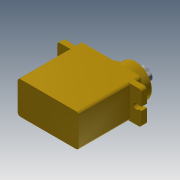
# Autodesk Inventor part: micro_servo
Saved by Autodesk Inventor 2015 (Build 190159000, 159)
## iProperties
Created: 2013-01-22
Part Number: micro_servo
Material: Generic
Document SubType Name: Modeling
Designer: idle-rug
Density: 1 g/cm^3
Appearance: Default
Author: idle-rug
Autodesk Inventor part; units mm, degrees
ref_plane "YZ Plane" through (0, 0, 0) normal (1, 0, 0) x (0, 1, 0)
ref_plane "XZ Plane" through (0, 0, 0) normal (0, 1, 0) x (-1, 0, 0)
ref_plane "XY Plane" through (0, 0, 0) normal (0, 0, 1) x (1, 0, 0)
sketch "Sketch1" plane through (0, 0, 0) normal (0, 1, 0) x (-1, 0, 0)
  line L0 (-11.6, -6.2) -> (11.6, -6.2)
  line L1 (11.6, -6.2) -> (11.6, 6.2)
  line L2 (11.6, 6.2) -> (-11.6, 6.2)
  line L3 (-11.6, 6.2) -> (-11.6, -6.2)
  line L4 (-11.6, -6.2) -> (11.6, 6.2) construction
  line L5 (11.6, -6.2) -> (-11.6, 6.2) construction
  point P0 (0, 0)
  constraints: 12 end point, 2 midpoint, 2 parallel, 1 horizontal, 1 perpendicular
extrude "Extrusion1" add sketch "Sketch1" along normal blind 31.7
sketch "Sketch2" plane through (11.6, 0, 6.2) normal (1, 0, 0) x (0, 0, -1)
  line L0 (12.4, 19.4) -> (0, 19.4)
  line L1 (0, 19.4) -> (0, 21.5)
  line L2 (0, 21.5) -> (12.4, 21.5)
  line L3 (12.4, 21.5) -> (12.4, 19.4)
  constraints: 8 end point
extrude "Extrusion2" add sketch "Sketch2" along normal blind 4.4
sketch "Sketch8" plane through (-11.6, 0, -6.2) normal (-1, 0, 0) x (0, 0, 1)
  line L0 (12.4, 19.4) -> (0, 19.4)
  line L1 (0, 19.4) -> (0, 21.5)
  line L2 (0, 21.5) -> (12.4, 21.5)
  line L3 (12.4, 21.5) -> (12.4, 19.4)
  point P0 (12.4, 0)
  point P1 (6.2, 0)
  constraints: 8 end point
extrude "Extrusion3" add sketch "Sketch8" along normal blind 4.4
sketch "Sketch10" plane through (0, 31.7, 0) normal (0, 1, 0) x (1, 0, 0)
  circle A0 centre (5.4, 0) radius 6.2
  constraints: 1 centre point
sketch "Sketch11" plane through (0, 31.7, 0) normal (0, 1, 0) x (1, 0, 0)
  circle A0 centre (-0.7, 0) radius 3.1
  point P0 (0, 0)
  constraints: 1 centre point
sketch "Sketch12" plane through (0, 31.7, 0) normal (0, 1, 0) x (1, 0, 0)
  line L0 (11.6, 6.2) -> (-11.6, 6.2) projected
  line L1 (-11.6, 6.2) -> (-11.6, -6.2) projected
  line L2 (-11.6, -6.2) -> (11.6, -6.2) projected
  line L3 (11.6, -6.2) -> (11.6, 6.2) projected
  point P0 (0, 0)
extrude "Extrusion4" cut sketch "Sketch12" against normal blind 7.9
extrude "Extrusion5" add sketch "Sketch10" against normal blind 7.9
extrude "Extrusion6" add sketch "Sketch11" against normal blind 7.9
sketch "Sketch13" plane through (0, 31.7, 0) normal (0, 1, 0) x (1, 0, 0)
  arc A0 (-0.0131, -3.0229) -> (-0.0131, 3.0229) centre (5.4, 0) ccw projected
  arc A1 (-0.0131, 3.0229) -> (-0.0131, -3.0229) centre (-0.7, 0) ccw projected
  circle A2 centre (5.4, 0) radius 4.75
  circle A3 centre (-0.7, 0) radius 1.35
  constraints: 2 centre point, 2 coincident
extrude "Extrusion7" cut sketch "Sketch13" against normal blind 4
sketch "Sketch14" plane through (5.4, 31.7, 0) normal (0, 1, 0) x (1, 0, 0)
  circle A0 centre (0, 0) radius 4.75 projected
  circle A1 centre (0, 0) radius 2.5
  point P0 (-4.75, 0)
  point P1 (-5.4, 0)
  dimension "d28" = 5
  constraints: 1 centre point, 1 coincident, 1 horizontal alignment
  measures "d28" diameter of A1
extrude "Extrusion8" cut sketch "Sketch14" against normal blind 3
sketch "Sketch15" plane through (-0.7, 31.7, 0) normal (0, 1, 0) x (1, 0, 0)
  circle A0 centre (0, 0) radius 1.35 projected
extrude "Extrusion9" cut sketch "Sketch15" against normal blind 3
sketch "Sketch16" plane through (11.6, 21.5, 6.2) normal (0, 1, 0) x (1, 0, 0)
  circle A0 centre (2.35, 6.2) radius 1.15
  line L0 (4.4, 6.2) -> (4.4, 5.5)
  line L1 (4.4, 5.5) -> (3.2624, 5.5)
  line L2 (4.4, 6.2) -> (4.4, 6.9)
  line L3 (4.4, 6.9) -> (3.2624, 6.9)
  point P0 (-11.6, 6.2)
  constraints: 8 end point, 2 point on circle, 1 centre point
sketch "Sketch17" plane through (-11.6, 21.5, 6.2) normal (0, 1, 0) x (1, 0, 0)
  circle A0 centre (-2.35, 6.2) radius 1.15
  line L0 (-4.4, 6.2) -> (-4.4, 6.9)
  line L1 (-4.4, 6.9) -> (-3.2624, 6.9)
  line L2 (-4.4, 6.2) -> (-4.4, 5.5)
  line L3 (-4.4, 5.5) -> (-3.2624, 5.5)
  point P0 (11.6, 6.2)
  constraints: 8 end point, 2 perpendicular, 2 point on circle, 1 centre point
sketch "Sketch18" plane through (-11.6, 21.5, 6.2) normal (0, 1, 0) x (1, 0, 0)
  point P0 (11.6, 6.2)
extrude "Extrusion10" cut sketch "Sketch17" against normal blind 3
extrude "Extrusion11" cut sketch "Sketch16" against normal blind 3
fillet "Fillet1" radius 1 1 edges at (-16, 20.45, -6.2)
sketch "Sketch20" plane through (-11.6, 21.5, 6.2) normal (0, 1, 0) x (1, 0, 0)
  point P0 (11.6, 6.2)
fillet "Fillet2" radius 1 1 edges at (16, 20.45, -6.2)
fillet "Fillet3" radius 1 1 edges at (-16, 20.45, 6.2)
fillet "Fillet4" radius 1 1 edges at (16, 20.45, 6.2)
fillet "Fillet5" radius 1 1 edges at (11.6, 22.65, 6.2)
fillet "Fillet6" radius 1 1 edges at (11.6, 22.65, -6.2)
fillet "Fillet7" radius 1 1 edges at (-11.6, 22.65, 6.2)
fillet "Fillet8" radius 1 1 edges at (-11.6, 22.65, -6.2)
fillet "Fillet9" radius 1 1 edges at (-11.6, 9.7, -6.2)
fillet "Fillet10" radius 1 1 edges at (11.6, 9.7, -6.2)
fillet "Fillet11" radius 1 1 edges at (11.6, 9.7, 6.2)
fillet "Fillet12" radius 1 1 edges at (-11.6, 9.7, 6.2)
body "Solid1"
